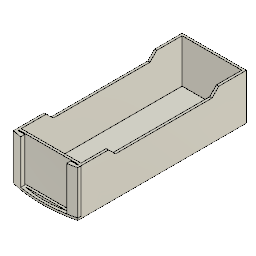
Res_Drawer v2 (Autodesk Fusion 360 design; units mm, degrees)
Autodesk Fusion 360 part; units mm, degrees
sketch "Boceto1" plane through (0, 0, 0) normal (0, 0, 1) x (1, 0, 0)
  line L0 (0, 72) -> (28, 72)
  line L1 (28, 72) -> (28, 0)
  line L2 (28, 0) -> (0, 0)
  line L3 (0, 0) -> (0, 72)
  dimension "d1" = 72
  dimension "d2" = 28
  constraint horizontal L0
  constraint vertical L1
  constraint horizontal L2
  constraint vertical L3
  constraint coincident L2.end L3.start
  measures "d1" distance of L0.end L1.end
  measures "d2" distance of L0.start L0.end
extrude "Extruir1" add sketch "Boceto1" along normal blind 1 makes body 1
sketch "Boceto2" plane through (0, 0, 0) normal (1, 0, 0) x (0, 1, 0)
  line L0 (0, 1) -> (0, 20)
  line L1 (0, 20) -> (12, 20)
  line L2 (12, 20) -> (15, 17)
  line L3 (15, 17) -> (57, 17)
  line L4 (57, 17) -> (60, 20)
  line L5 (60, 20) -> (72, 20)
  line L6 (72, 20) -> (72, 1)
  line L7 (72, 1) -> (0, 1)
  line L8 (0, 1) -> (72, 1)
  dimension "d5" = 19
  dimension "d6" = 12
  dimension "d7" = 12
  dimension "d8" = 72
  dimension "d9" = 45
  dimension "d12" = 16
  constraint vertical L0
  constraint perpendicular L0 L1
  constraint perpendicular L0 L3
  constraint perpendicular L2 L4
  constraint parallel L3 L5
  constraint perpendicular L5 L6
  constraint perpendicular L0 L7
  constraint coincident L0.start L7.end
  constraint collinear L1 L5
  measures "d5" distance of L0.start L0.end
  measures "d6" distance of L0.end L1.end
  measures "d7" distance of L4.end L5.end
  measures "d8" distance of L0 L6
  measures "d9" angle of L1 L2
  measures "d12" distance of L3 L7
extrude "Extruir2" add sketch "Boceto2" along normal blind 28 bodies 1
shell "Vaciado1" thickness 1 removed faces 5 at (9.3333, 4, 20) at (9.3333, 13, 19) at (9.3333, 29, 17) at (9.3333, 58, 18) at (9.3333, 64, 20) on bodies 1
sketch "Boceto5" plane through (0, 0, 0) normal (0, 0, -1) x (1, 0, 0)
  line L0 (28, 0) -> (0, 0)
  line L1 (0, 0) -> (0, -72)
  line L2 (0, -72) -> (28, -72)
  line L3 (28, -72) -> (28, 0)
  line L4 (0, 0) -> (0, 1.4)
  line L5 (28, 0) -> (28, 1.4)
  arc A0 (28, 1.4) -> (0, 1.4) centre (14, -56.9438) ccw
  line L6 (0, 0) -> (28, 0)
  dimension "d28" = 1.4
  dimension "d29" = 1.4
  dimension "d30" = 60
  constraint coincident L0.end L1.start
  constraint perpendicular L0 L4
  constraint coincident L0.start L3.end
  constraint perpendicular L0 L5
  measures "d28" distance of L0.end L4.end
  measures "d29" distance of L0.start L5.end
  measures "d30" radius of A0
extrude "Extruir3" add sketch "Boceto5" against normal blind 1 separate body contours L0 L4 L5 A0 L6 makes body 2
sketch "Boceto6" plane through (0, 0, 1) normal (0, 0, 1) x (-1, 0, 0)
  line L0 (-28, 0) -> (0, 0)
  line L1 (0, 0) -> (0, 1.4)
  arc A0 (0, 1.4) -> (-28, 1.4) centre (-14, -56.9438) ccw
  line L2 (-28, 1.4) -> (-28, 0)
  line L3 (-5, 1) -> (-23, 1)
  arc A1 (-5, 1) -> (-23, 1) centre (-14, -37.9744) ccw
  line L4 (0, 0) -> (-28, 0)
  dimension "d35" = 18
  dimension "d36" = 5
  dimension "d37" = 40
  dimension "d38" = 1
  constraint parallel L0 L3
  measures "d35" distance of L3.start L3.end
  measures "d36" distance of L1 L3.start
  measures "d37" radius of A1
  measures "d38" distance of L3.start L4
extrude "Extruir4" cut sketch "Boceto6" against normal blind 1 contours L3 A1 bodies 2
sketch "Boceto7" plane through (0, 0, 1) normal (0, 0, 1) x (-1, 0, 0)
  line L0 (-5, 1) -> (-23, 1)
  arc A0 (-5, 1) -> (-23, 1) centre (-14, -37.9744) ccw
  line L1 (-28, 0) -> (0, 0)
  line L2 (0, 0) -> (0, 1.4)
  arc A1 (0, 1.4) -> (-28, 1.4) centre (-14, -56.9438) ccw
  line L3 (-28, 1.4) -> (-28, 0)
  line L4 (-1, 0) -> (0, 0)
  line L5 (-4, 2.217) -> (-4, 0.4)
  line L6 (-4, 0.4) -> (-1, 0.4)
  line L7 (-1, 0.4) -> (-1, 0)
  arc A2 (0, 1.4) -> (-4, 2.217) centre (-14, -56.9438) ccw
  line L8 (-14, -72) -> (-14, 0) construction
  line L9 (-24, 0.4) -> (-27, 0.4)
  line L10 (-27, 0.4) -> (-27, 0)
  line L11 (-27, 0) -> (-28, 0)
  line L12 (-28, 0) -> (-28, 1.4)
  arc A3 (-24, 2.217) -> (-28, 1.4) centre (-14, -56.9438) ccw
  line L13 (-24, 2.217) -> (-24, 0.4)
  dimension "d39" = 0.4
  dimension "d40" = 1
  dimension "d41" = 4
  dimension "d42" = 60
  constraint coincident L1.end L2.start
  constraint coincident A1 L5.start
  constraint perpendicular L1 L5
  constraint perpendicular L5 L6
  constraint coincident L1 L4.start
  constraint perpendicular L6 L7
  constraint coincident L2.end A1.start
  constraint midpoint L1 L8.end
  constraint symmetric L1.end L8 L1.start
  constraint symmetric L2.end L8 A1.end
  constraint symmetric L5.start L8 A3.start
  constraint symmetric L5.end L8 L9.start
  constraint symmetric L6.end L8 L9.end
  constraint symmetric L4.start L8 L10.end
  constraint symmetric A2 L8 A3
  measures "d39" distance of L6.end L4.start
  measures "d40" distance of L1.end L4.start
  measures "d41" distance of L2 L5
  measures "d42" radius of A2
extrude "Extruir5" add sketch "Boceto7" along normal blind 19 contours L1 A1 L3 L9 L10 L11 L12 A3 L13 | L1 L2 A1 L4 L5 L6 L7 A2 bodies 1 2
equation "d1 = internal_depth + 2 mm"
equation "d2 = internal_width + 2 mm"
equation "d5 = internal_height"
equation "d6 = ( internal_depth + 2 mm ) / 6"
equation "d7 = ( internal_depth + 2 mm ) / 6"
equation "d8 = internal_depth + 2 mm"
equation "d12 = internal_height - 3 mm"
equation "internal_depth = 70 mm"
equation "internal_width = 26 mm"
equation "internal_height = 19 mm"
equation "wall_width = 1 mm"
equation "d24 = wall_width"
equation "d35 = ( internal_width + 2 mm ) - 10 mm"
equation "d43 = internal_height"
